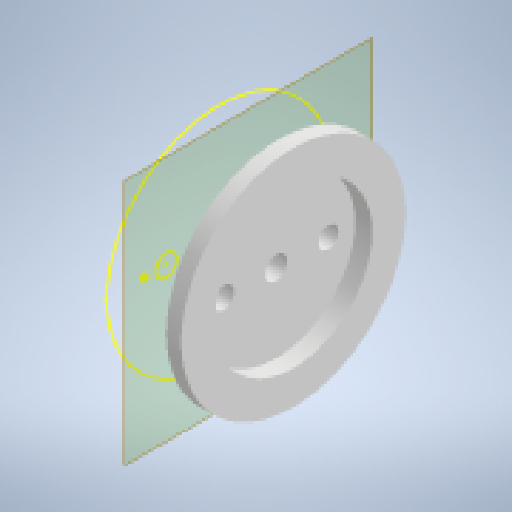
# Autodesk Inventor part: bubinek_BOTTOM
Saved by Autodesk Inventor 2023.1 (Build 271208000, 208)
## iProperties
Created: 2022-11-11
Part Number: bubinek_BOTTOM
Material: Všeobecné
Document SubType Name: Modeling
Designer: zavrel
Density: 1 g/cm^3
Appearance: Výchozí
Author: zavrel
Autodesk Inventor part; units mm, degrees
ref_plane "YZ Plane" through (0, 0, 0) normal (1, 0, 0) x (0, 1, 0)
ref_plane "XZ Plane" through (0, 0, 0) normal (0, 1, 0) x (-1, 0, 0)
ref_plane "XY Plane" through (0, 0, 0) normal (0, 0, 1) x (1, 0, 0)
sketch "Náčrt1" plane through (0, 0, 0) normal (0, 1, 0) x (-1, 0, 0)
  line L0 (0, 0) -> (0, -15)
  line L1 (10, 0) -> (10, -15)
  line L2 (6, -5) -> (4, -5)
  line L3 (10, -15) -> (0, -15)
  line L4 (6, -5) -> (8, 0)
  line L5 (8, 0) -> (10, 0)
  line L6 (4, -5) -> (2, 0)
  line L7 (2, 0) -> (0, 0)
  dimension "d0" = 2
  dimension "d1" = 5
  dimension "d2" = 15
  dimension "d5" = 2
  dimension "d6" = 10
  constraints: 16 end point, 3 equal length, 3 horizontal, 2 vertical, 1 collinear, 1 horizontal alignment, 1 point on line
  measures "d0" distance of L2.start L2.end
  measures "d1" distance from line of L0.start L2
  measures "d2" distance of L1.start L1.end
  measures "d5" distance of L6.end L0.start
  measures "d6" distance between parallel lines of L0 L1
revolve "Rotace1" add sketch "Náčrt1" angle 360 about axis through (-10, 0, -15) along (1, 0, 0)
sketch "Náčrt2" plane through (0, 0, -15) normal (1, 0, 0) x (0, 0, -1)
  circle A0 centre (0, 0) radius 15 projected
  circle A1 centre (0, 0) radius 10 projected
  circle A2 centre (0, 0) radius 10.5
  point P0 (-15, 0)
  dimension "d8" = 21
  constraints: 1 centre point, 1 coincident
  measures "d8" diameter of A2
extrude "Vysunutí1" cut sketch "Náčrt2" against normal blind 2.3 contours A1 | A2
sketch "Náčrt3" plane through (-10, 0, -15) normal (-1, 0, 0) x (0, 0, 1)
  circle A0 centre (0, 0) radius 15 projected
  circle A1 centre (0, 0) radius 3
  point P0 (15, 0)
  dimension "d11" = 6
  constraints: 1 centre point, 1 coincident
  measures "d11" diameter of A1
extrude "Vysunutí2" cut sketch "Náčrt3" against normal blind 3 contours A1
sketch "Náčrt4" plane through (-7, 0, -15) normal (-1, 0, 0) x (0, 0, 1)
  circle A0 centre (0, 0) radius 15 projected
  circle A1 centre (0, 0) radius 10 projected
  circle A2 centre (0, 0) radius 1.5
  point P0 (15, 0)
  dimension "d14" = 3
  constraints: 1 centre point, 1 coincident
  measures "d14" diameter of A2
extrude "Vysunutí3" cut sketch "Náčrt4" against normal through all contours A2
sketch "Náčrt5" plane through (-10, 0, -15) normal (-1, 0, 0) x (0, 0, 1)
  circle A0 centre (0, 0) radius 3 projected
  circle A1 centre (0, 0) radius 15 projected
  circle A2 centre (0, 0) radius 1.5 construction
  circle A3 centre (0, 0) radius 7 construction
  circle A4 centre (7, 0) radius 1.4
  circle A5 centre (0, 0) radius 10 construction
  circle A6 centre (10, 0) radius 0.5
  circle A7 centre (0, 0) radius 15 construction
  line L0 (0, 15) -> (0, -15) construction
  circle A8 centre (-7, 0) radius 1.4
  point P0 (15, 0)
  dimension "d17" = 8
  dimension "d18" = 2.8
  dimension "d21" = 5
  dimension "d22" = 1
  constraints: 3 centre point, 2 coincident, 2 end point, 2 horizontal alignment, 2 point on circle, 1 symmetric about line, 1 vertical, 5 other
  measures "d18" diameter of A4
  measures "d22" diameter of A6
extrude "Vysunutí4" cut sketch "Náčrt5" against normal through all contours A4 | A6 | A8
sketch "Náčrt6" plane through (-10, 0, -15) normal (-1, 0, 0) x (0, 0, 1)
  circle A0 centre (7, 0) radius 1.4 projected
  circle A1 centre (10, 0) radius 0.5 projected
  circle A2 centre (0, 0) radius 3 projected
  circle A3 centre (0, 0) radius 15 projected
  point P0 (15, 0)
ref_plane "Pracovní rovina1" through (-6, 0, -15) normal (-1, 0, 0) x (0, 0, 1)
split "Rozdělit1" plane through (-6, 0, -15) removes the side toward (-1, 0, 0)
sketch "Sketch7" plane through (-6, 0, -15) normal (-1, 0, 0) x (0, 0, 1)
  circle A0 centre (-7, 0) radius 1.5 projected
  circle A1 centre (7, 0) radius 1.4 projected
  arc A2 (9.9875, 0.4998) -> (9.9875, -0.4998) centre (10, 0) ccw projected
  arc A3 (9.9875, 0.4998) -> (9.9875, -0.4998) centre (0, 0) ccw projected
  circle A4 centre (0, 0) radius 1.5 projected
  point P0 (15, 0)
extrude "Extrusion5" cut sketch "Sketch7" against normal blind 1 contours A0 | A1 | A2 A3 | A4
